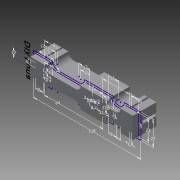
# Autodesk Inventor part: Spirulina_prototype2
Saved by Autodesk Inventor 2015 (Build 190159000, 159)
## iProperties
Created: 2015-05-18
Part Number: Spirulina_prototype2
Material: Generic
Document SubType Name: Modeling
Designer: Openlab
Density: 1 g/cm^3
Appearance: Default
Author: Openlab
Autodesk Inventor part; units mm, degrees
ref_plane "YZ Plane" through (0, 0, 0) normal (1, 0, 0) x (0, 1, 0)
ref_plane "XZ Plane" through (0, 0, 0) normal (0, 1, 0) x (-1, 0, 0)
ref_plane "XY Plane" through (0, 0, 0) normal (0, 0, 1) x (1, 0, 0)
sketch "Sketch1" plane through (0, 0, 0) normal (0, 1, 0) x (-1, 0, 0)
  line L0 (45.05, -5.25) -> (32.55, -5.25)
  line L1 (32.55, -5.25) -> (32.55, -17.75)
  line L2 (32.55, -17.75) -> (45.05, -17.75)
  line L3 (45.05, -17.75) -> (45.05, -5.25)
  line L4 (0, 0) -> (0, -23)
  line L5 (112.6, -23) -> (112.6, 0)
  line L6 (77.3838, -11.5) -> (49.3838, -11.5) construction
  line L7 (38.8, -2.0322) -> (38.8, -23.0322) construction
  line L8 (93.8, -8.9) -> (112.6, -8.9)
  line L9 (112.6, -14.1) -> (93.8, -14.1)
  line L10 (9.8, 0) -> (9.8, -23)
  line L11 (8, 0) -> (8, -23)
  line L12 (24.8, -10) -> (0, -10)
  line L13 (24.8, -13) -> (0, -13)
  line L14 (102.8, -14.55) -> (101.3, -14.55)
  line L15 (101.3, -14.55) -> (101.3, -8.45)
  line L16 (101.3, -8.45) -> (102.8, -8.45)
  line L17 (50.8, -10) -> (50.8, -13)
  line L18 (50.8, -13) -> (45.05, -13)
  line L19 (45.05, -10) -> (50.8, -10)
  line L20 (32.55, -13) -> (26.8, -13)
  line L21 (26.8, -10) -> (32.55, -10)
  line L22 (102.8, -17.5) -> (100.8, -17.5)
  line L23 (100.8, -17.5) -> (100.8, -15.5)
  line L24 (100.8, -15.5) -> (102.8, -15.5)
  line L25 (102.8, -7.5) -> (100.8, -7.5)
  line L26 (100.8, -7.5) -> (100.8, -5.5)
  line L27 (100.8, -5.5) -> (102.8, -5.5)
  line L28 (137, -16.5) -> (122.5716, -16.5) construction
  line L29 (137, -6.5) -> (123, -6.5) construction
  line L30 (104.6, -17.5) -> (106.6, -17.5)
  line L31 (106.6, -17.5) -> (106.6, -15.5)
  line L32 (106.6, -15.5) -> (104.6, -15.5)
  line L33 (104.6, -7.5) -> (106.6, -7.5)
  line L34 (106.6, -7.5) -> (106.6, -5.5)
  line L35 (106.6, -5.5) -> (104.6, -5.5)
  line L36 (104.6, -23) -> (104.6, -17.5)
  line L37 (102.8, -17.5) -> (102.8, -23)
  line L38 (104.6, -15.5) -> (104.6, -7.5)
  line L39 (104.6, -5.5) -> (104.6, 0)
  line L40 (102.8, 0) -> (102.8, -5.5)
  line L41 (102.8, -7.5) -> (102.8, -15.5)
  line L42 (45.05, -17.75) -> (53.25, -17.75)
  line L43 (53.25, -17.75) -> (53.25, -14.55)
  line L44 (53.25, -14.55) -> (45.05, -14.55)
  line L45 (45.05, -8.45) -> (53.25, -8.45)
  line L46 (53.25, -8.45) -> (53.25, -5.25)
  line L47 (53.25, -5.25) -> (45.05, -5.25)
  line L48 (48.05, -17.75) -> (48.05, -14.55)
  line L49 (50.05, -17.75) -> (50.05, -14.55)
  line L50 (50.05, -8.45) -> (50.05, -5.25)
  line L51 (48.05, -8.45) -> (48.05, -5.25)
  line L52 (52.8, -10) -> (52.8, -13)
  line L53 (26.8, -10) -> (26.8, -13)
  line L54 (24.8, -10) -> (24.8, -13)
  line L55 (52.8, -13) -> (91.6763, -13)
  line L56 (52.8, -10) -> (91.6763, -10)
  arc A0 (93.8, -8.9) -> (91.6763, -10) centre (93.8, -11.5) ccw
  arc A1 (91.6763, -13) -> (93.8, -14.1) centre (93.8, -11.5) ccw
  arc A2 (96.8, -23) -> (90.8, -17) centre (90.8, -23) ccw
  arc A3 (63.25, -17) -> (57.25, -23) centre (63.25, -23) ccw
  arc A4 (90.8, -6) -> (96.8, 0) centre (90.8, 0) ccw
  arc A5 (57.25, 0) -> (63.25, -6) centre (63.25, 0) ccw
  line L57 (90.8, -17) -> (63.25, -17)
  line L58 (90.8, -6) -> (63.25, -6)
  line L59 (112.6, 0) -> (96.8, 0)
  line L60 (96.8, -23) -> (112.6, -23)
  arc A6 (29.55, -23) -> (23.55, -17) centre (23.55, -23) ccw
  arc A7 (23.55, -6) -> (29.55, 0) centre (23.55, 0) ccw
  arc A8 (19.55, -17) -> (13.55, -23) centre (19.55, -23) ccw
  arc A9 (13.55, 0) -> (19.55, -6) centre (19.55, 0) ccw
  line L61 (23.55, -6) -> (19.55, -6)
  line L62 (23.55, -17) -> (19.55, -17)
  line L63 (0, -23) -> (13.55, -23)
  line L64 (29.55, -23) -> (57.25, -23)
  line L65 (57.25, 0) -> (29.55, 0)
  line L66 (13.55, 0) -> (0, 0)
  line L67 (115.3, -25) -> (115.3, 2)
  line L68 (-2.7, 2) -> (-2.7, -25)
  arc A10 (65.25, -19) -> (59.25, -25) centre (65.25, -25) ccw
  arc A11 (94.8, -25) -> (88.8, -19) centre (88.8, -25) ccw
  line L69 (56.3, -20.25) -> (56.3, -1) construction
  arc A12 (59.25, 2) -> (65.25, -4) centre (65.25, 2) ccw
  arc A13 (88.8, -4) -> (94.8, 2) centre (88.8, 2) ccw
  arc A14 (15.55, 2) -> (27.55, 2) centre (21.55, 2) ccw
  arc A15 (27.55, -25) -> (15.55, -25) centre (21.55, -25) ccw
  line L70 (88.8, -19) -> (65.25, -19)
  line L71 (88.8, -4) -> (65.25, -4)
  line L72 (115.3, 2) -> (94.8, 2)
  line L73 (94.8, -25) -> (115.3, -25)
  line L74 (-2.7, -25) -> (15.55, -25)
  line L75 (27.55, -25) -> (59.25, -25)
  line L76 (59.25, 2) -> (27.55, 2)
  line L77 (15.55, 2) -> (-2.7, 2)
  line L78 (125.6323, 7.0516) -> (125.6323, -28.0034) construction
  line L79 (125.6323, -28.0034) -> (118.769, -28.0034) construction
  line L80 (118.769, -28.0034) -> (118.769, 7.0516) construction
  line L81 (118.769, 7.0516) -> (125.6323, 7.0516) construction
  point P0 (104.6, -8.9)
  point P1 (104.6, -14.1)
  point P2 (102.8, -8.9)
  point P3 (102.8, -14.1)
  point P4 (9.8, -13)
  point P5 (8, -13)
  point P6 (8, -10)
  point P7 (9.8, -10)
  point P8 (38.8, -11.5)
  point P9 (101.3, -14.1)
  point P10 (101.3, -8.9)
  dimension "d0" = 12.5
  dimension "d1" = 12.5
  dimension "d3" = 23
  dimension "d12" = 5.2
  dimension "d20" = 1.8
  dimension "d25" = 3
  dimension "d36" = 6.1
  dimension "d37" = 1.5
  dimension "d62" = 3
  dimension "d63" = 3
  dimension "d94" = 2
  dimension "d95" = 2
  dimension "d96" = 10
  dimension "d97" = 1.8
  dimension "d106" = 8.2
  dimension "d107" = 3
  dimension "d108" = 2
  dimension "d109" = 3.2
  dimension "d113" = 1.5
  dimension "d114" = 2
  dimension "d115" = 64
  dimension "d116" = 29
  dimension "d117" = 8
  dimension "d118" = 8
  dimension "d119" = 2
  dimension "d120" = 12
  dimension "d121" = 12
  dimension "d122" = 9
  dimension "d129" = 12
  dimension "d130" = 12
  dimension "d131" = 10
  dimension "d134" = 9
  dimension "d135" = 4
  dimension "d149" = 118
  dimension "d150" = 27
  dimension "d152" = 11
  dimension "d153" = 12
  dimension "d154" = 14
  constraints: 156 end point, 69 point on line, 63 perpendicular, 32 point on circle, 26 parallel, 21 collinear, 17 horizontal, 16 centre point, 14 tangent, 13 equal radius, 7 vertical alignment, 3 vertical, 1 coincident, 18 other
  measures "d0" distance of L2.end L1.end
  measures "d1" distance of L0.end L1.end
  measures "d3" distance of L4.end L4.start
  measures "d12" distance between parallel lines of L9 L8
  measures "d20" distance between parallel lines of L11 L10
  measures "d25" distance between parallel lines of L13 L12
  measures "d36" distance of L14.end L15.end
  measures "d37" distance of L14.start L14.end
  measures "d62" distance between parallel lines of L19 L18
  measures "d63" distance between parallel lines of L21 L20
  measures "d94" distance of L22.end L23.end
  measures "d95" distance of L22.start L22.end
  measures "d96" distance between parallel lines of L29 L28
  measures "d97" distance between parallel lines of L40 L39
  measures "d106" distance of L2.end L42.end
  measures "d107" distance between parallel lines of L48 L3
  measures "d108" distance between parallel lines of L48 L49
  measures "d109" distance of L42.end L43.end
  measures "d113" distance of L15.end L16.end
  measures "d114" distance between parallel lines of L52 L17
  measures "d115" distance between parallel lines of L37 L7
  measures "d116" distance between parallel lines of L10 L7
  measures "d117" distance between parallel lines of L4 L11
  measures "d118" distance between parallel lines of L5 L36
  measures "d119" distance between parallel lines of L54 L53
  measures "d120" distance between parallel lines of L53 L7
  measures "d121" distance between parallel lines of L17 L7
  measures "d122" distance from line of A0.centre L41
  measures "d129" diameter of A4
  measures "d130" distance from line of L40 A4.centre
  measures "d131" distance from line of A5.centre L46
  measures "d134" distance from line of A6.centre L1
  measures "d135" distance of A8.centre A6.centre
  measures "d149" distance of L68.end L67.start
  measures "d150" distance of L68.start L68.end
  measures "d152" distance from line of A14.centre L1
  measures "d153" distance from line of A12.centre L46
  measures "d154" distance from line of A13.centre L40
extrude "Extrusion16" add sketch "Sketch1" against normal blind 6 contours L3 L2 L1 L0 | L47 L51 L45 L3 | L47 L50 L45 L51 | L1 L20 L53 L21 | L19 L17 L18 L3 | L47 L46 L45 L50 | L44 L48 L42 L3 | L44 L49 L42 L48 | L44 L43 L42 L49 | L66 L11 L12 L4 | L12 L11 L13 L4 | L66 L10 L12 L11 | L13 L11 L63 L4 | L12 L10 L13 L11 | L66 A9 L61 A7 L65 A5 L58 A4 L59 L40 L27 L26 L25 L41 L16 L15 L8 A0 L56 L52 L55 A1 L9 L14 L24 L23 L22 L37 L60 A2 L57 A3 L64 A6 L62 A8 L63 L10 L13 L54 L12 | L13 L10 L63 L11 | L12 L54 L13 L10 | L59 L39 L35 L34 L33 L38 L8 L41 L25 L26 L27 L40 | L59 L5 L8 L38 L33 L34 L35 L39 | L37 L22 L23 L24 L41 L9 L38 L32 L31 L30 L36 L60 | L5 L9 L38 L8 | L36 L30 L31 L32 L38 L9 L5 L60 | L38 L9 L41 L8 | L41 L8 L15 L16 | L41 L9 L15 L8 | L41 L14 L15 L9 | L15 L9 A1 L55 L52 L56 A0 L8
extrude "Extrusion17" add sketch "Sketch1" along normal blind 20 contours L66 L11 L12 L4 | L13 L11 L63 L4 | L66 A9 L61 A7 L65 A5 L58 A4 L59 L40 L27 L26 L25 L41 L16 L15 L8 A0 L56 L52 L55 A1 L9 L14 L24 L23 L22 L37 L60 A2 L57 A3 L64 A6 L62 A8 L63 L10 L13 L54 L12 | L59 L5 L8 L38 L33 L34 L35 L39 | L36 L30 L31 L32 L38 L9 L5 L60
extrude "Extrusion18" add sketch "Sketch1" along normal blind 5 contours L1 L20 L53 L21 | L19 L17 L18 L3 | L12 L11 L13 L4 | L12 L54 L13 L10 | L5 L9 L38 L8 | L15 L9 A1 L55 L52 L56 A0 L8
extrude "Extrusion19" add sketch "Sketch1" along normal blind 9 contours L47 L50 L45 L51 | L44 L49 L42 L48
sketch "Sketch2" plane through (0, -6, 0) normal (1, 0, 0) x (0, 0, -1)
  line L0 (11.5, 16) -> (11.5, 6.397) construction
  line L1 (0, 6) -> (23, 6) construction
  line L2 (0, 1.5617) -> (0, -5) construction
  line L3 (23, -1.6862) -> (23, -8) construction
  point P0 (11.5, 16)
  dimension "d139" = 10
  constraints: 6 end point, 3 point on line, 3 vertical, 1 other
  measures "d139" distance from line of L1 point (11.5, 16)
hole "Hole1" at (0, 10, -11.5) direction (-1, 0, 0) diameter 2 end through all
body "Solid4"
